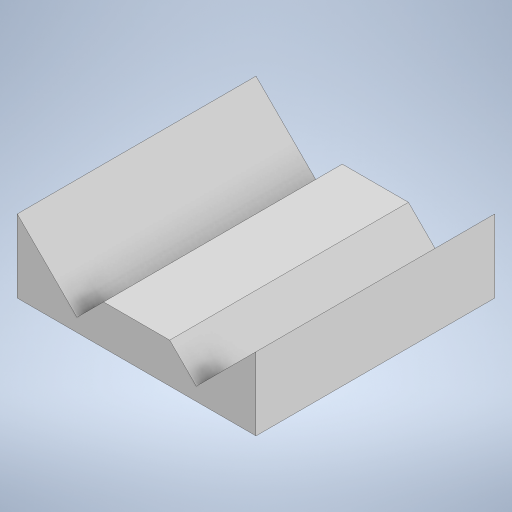
# Autodesk Inventor part: Drone Charging Base
Saved by Autodesk Inventor 2023 (Build 270158000, 158)
## iProperties
Created: 2022-12-15
Part Number: Drone Charging Base
Material: Generic
Document SubType Name: Modeling
Designer: chase
Density: 1 g/cm^3
Appearance: Default
Author: chase
Autodesk Inventor part; units mm, degrees
ref_plane "YZ Plane" through (0, 0, 0) normal (1, 0, 0) x (0, 1, 0)
ref_plane "XZ Plane" through (0, 0, 0) normal (0, 1, 0) x (-1, 0, 0)
ref_plane "XY Plane" through (0, 0, 0) normal (0, 0, 1) x (1, 0, 0)
sketch "Sketch1" plane through (0, 0, 0) normal (0, 0, 1) x (1, 0, 0)
  line L0 (0, 0) -> (914.4, 0)
  line L1 (914.4, 0) -> (914.4, 279.0857)
  line L2 (787.7143, 152.4) -> (126.6857, 152.4)
  line L3 (0, 279.0857) -> (0, 0)
  line L4 (457.2, 0) -> (457.2, 152.4)
  line L5 (685.8, 0) -> (685.8, 152.4)
  line L6 (228.6, 0) -> (228.6, 152.4)
  line L7 (228.6, 50.4857) -> (-130.6102, 409.6959)
  line L8 (228.6, 50.4857) -> (330.5143, 152.4)
  line L9 (685.8, 50.4857) -> (583.8857, 152.4)
  line L10 (685.8, 50.4857) -> (1045.0102, 409.6959)
  line L11 (330.2, 0) -> (330.2, 152.0857)
  line L12 (127, 0) -> (127, 152.4)
  line L13 (584.2, 0) -> (584.2, 152.0857)
  line L14 (787.4, 0) -> (787.4, 152.4)
  point P0 (330.2, 152.4)
  dimension "d18" = 101.6
  dimension "d19" = 101.6
  dimension "d20" = 101.6
  dimension "d21" = 101.6
  constraints: 28 end point, 9 point on line, 7 parallel, 2 horizontal, 1 midpoint, 1 perpendicular, 12 other
  measures "d18" distance between parallel lines of L6 L11
  measures "d19" distance between parallel lines of L6 L12
  measures "d20" distance between parallel lines of L5 L13
  measures "d21" distance between parallel lines of L5 L14
extrude "Extrusion1" add sketch "Sketch1" against normal blind 914.4 contours L3 L7 L12 L0 | L12 L7 L6 L0 | L6 L8 L11 L0 | L11 L8 L2 L4 L0 | L4 L2 L9 L13 L0 | L13 L9 L5 L0 | L5 L10 L14 L0 | L14 L10 L1 L0
body "Solid1"
